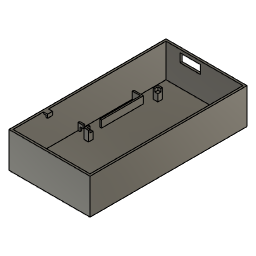
casing (Autodesk Fusion 360 design; units mm, degrees)
Autodesk Fusion 360 part; units mm, degrees
sketch "Sketch1" plane through (0, 0, 0) normal (0, 0, 1) x (1, 0, 0)
  line L0 (-40, 77.5) -> (40, 77.5)
  line L1 (40, 77.5) -> (40, -77.5)
  line L2 (40, -77.5) -> (-40, -77.5)
  line L3 (-40, -77.5) -> (-40, 77.5)
  dimension "d5" = 80
  dimension "d6" = 40
  dimension "d7" = 155
  dimension "d8" = 77.5
  constraint horizontal L0
  constraint vertical L1
  constraint horizontal L2
  constraint vertical L3
  measures "d5" distance of L0.start L0.end
  measures "d6" horizontal distance of origin L0.start
  measures "d7" distance of L0.start L2.end
  measures "d8" vertical distance of origin L0.start
extrude "Extrude1" add sketch "Sketch1" along normal blind 35
shell "Shell1" thickness 2 removed faces 1 at (-13.3333, -25.8333, 35)
sketch "Sketch2" plane through (0, 0, 2) normal (0, 0, 1) x (-1, 0, 0)
  line L0 (38, 75.5) -> (-38, 75.5)
  line L1 (-38, 75.5) -> (-38, -75.5)
  line L2 (-38, -75.5) -> (38, -75.5)
  line L3 (38, -75.5) -> (38, 75.5)
  line L4 (26, -55.5) -> (-24, -55.5)
  line L5 (-24, -55.5) -> (-24, 14.5)
  line L6 (-24, 14.5) -> (26, 14.5)
  line L7 (26, 14.5) -> (26, -55.5)
  line L8 (38, -42.2) -> (30, -42.2)
  line L9 (30, -42.2) -> (30, 9.8)
  line L10 (30, 9.8) -> (38, 9.8)
  line L11 (38, 9.8) -> (38, -42.2)
  line L12 (-28, -75) -> (-33, -75)
  line L13 (-33, -75) -> (-33, 35)
  line L14 (-33, 35) -> (-28, 35)
  line L15 (-28, 35) -> (-28, -75)
  line L16 (-24, 42) -> (-37, 42)
  line L17 (-37, 42) -> (-37, 72)
  line L18 (-37, 72) -> (-24, 72)
  line L19 (-24, 72) -> (-24, 42)
  spline S0 degree 5 poles (-24, 42) (-24.0273, 41.9316) (-24.0869, 41.788) (-24.1914, 41.5521) (-24.3612, 41.196) (-24.6275, 40.6777) (-24.9511, 40.0815) (-25.3338, 39.405) (-25.7728, 38.652) (-26.2629, 37.8296) (-26.7987, 36.9452) (-27.2602, 36.1929) (-27.6235, 35.6054) (-27.8733, 35.2035) (-28, 35) knots 0 0 0 0 0 0 0.1 0.2 0.3 0.4 0.5 0.6 0.7 0.8 0.9 1 1 1 1 1 1
  spline S1 degree 5 poles (-33, 35) (-33.1102, 35.2086) (-33.3283, 35.6201) (-33.648, 36.2209) (-34.0595, 36.9881) (-34.547, 37.8867) (-35.005, 38.718) (-35.4298, 39.4743) (-35.8182, 40.1481) (-36.1686, 40.7356) (-36.4823, 41.24) (-36.7056, 41.5808) (-36.8584, 41.8031) (-36.9539, 41.9368) (-37, 42) knots 0 0 0 0 0 0 0.1 0.2 0.3 0.4 0.5 0.6 0.7 0.8 0.9 1 1 1 1 1 1
  line L20 (-24, 72) -> (0, 72)
  line L21 (0, 72) -> (0, 59)
  line L22 (0, 59) -> (-24, 59)
  line L23 (-24, 59) -> (-24, 72)
  line L24 (0, 62.45) -> (7.5, 62.45)
  line L25 (7.5, 62.45) -> (7.5, 68.55)
  line L26 (7.5, 68.55) -> (0, 68.55)
  line L27 (0, 68.55) -> (0, 62.45)
  line L28 (7.5, 72.95) -> (7.5, 62.45)
  line L29 (7.5, 61.75) -> (11.5, 61.75)
  line L30 (11.5, 61.75) -> (11.5, 69.25)
  line L31 (11.5, 69.25) -> (7.5, 69.25)
  line L32 (7.5, 69.25) -> (7.5, 61.75)
  line L33 (-26.5, -75.5) -> (-28, -75.5)
  line L34 (-28, -75.5) -> (-28, 24.5)
  line L35 (-28, 24.5) -> (-26.5, 24.5)
  line L36 (-26.5, 24.5) -> (-26.5, -75.5)
  line L37 (-33, -75.5) -> (-34.5, -75.5)
  line L38 (-34.5, -75.5) -> (-34.5, 24.5)
  line L39 (-34.5, 24.5) -> (-33, 24.5)
  line L40 (-33, 24.5) -> (-33, -75.5)
  line L41 (-24, 59) -> (1.5, 59)
  line L42 (1.5, 59) -> (1.5, 57.5)
  line L43 (1.5, 57.5) -> (-24, 57.5)
  line L44 (-24, 57.5) -> (-24, 59)
  line L45 (0, 59) -> (1.5, 59)
  line L46 (1.5, 59) -> (1.5, 61)
  line L47 (1.5, 61) -> (0, 61)
  line L48 (0, 61) -> (0, 59)
  line L49 (-24, 57.5) -> (-22.5, 57.5)
  line L50 (-22.5, 57.5) -> (-22.5, 45)
  line L51 (-22.5, 45) -> (-24, 45)
  line L52 (-24, 45) -> (-24, 57.5)
  line L53 (26, -55.5) -> (23, -55.5)
  line L54 (23, -55.5) -> (23, -52.5)
  line L55 (23, -52.5) -> (26, -52.5)
  line L56 (26, -52.5) -> (26, -55.5)
  line L57 (-24, -55.5) -> (-21, -55.5)
  line L58 (-21, -55.5) -> (-21, -52.5)
  line L59 (-21, -52.5) -> (-24, -52.5)
  line L60 (-24, -52.5) -> (-24, -55.5)
  line L61 (23, -55.5) -> (26, -55.5)
  line L62 (26, -55.5) -> (26, -57)
  line L63 (26, -57) -> (23, -57)
  line L64 (23, -57) -> (23, -55.5)
  line L65 (26, -57) -> (27.5, -57)
  line L66 (27.5, -57) -> (27.5, -52.5)
  line L67 (27.5, -52.5) -> (26, -52.5)
  line L68 (26, -52.5) -> (26, -57)
  line L69 (-21, -55.5) -> (-24, -55.5)
  line L70 (-24, -55.5) -> (-24, -57)
  line L71 (-24, -57) -> (-21, -57)
  line L72 (-21, -57) -> (-21, -55.5)
  line L73 (-24, -57) -> (-25.5, -57)
  line L74 (-25.5, -57) -> (-25.5, -52.5)
  line L75 (-25.5, -52.5) -> (-24, -52.5)
  line L76 (-24, -52.5) -> (-24, -57)
  line L77 (38, -42.2) -> (28.5, -42.2)
  line L78 (28.5, -42.2) -> (28.5, -43.7)
  line L79 (28.5, -43.7) -> (38, -43.7)
  line L80 (38, -43.7) -> (38, -42.2)
  line L81 (30, -42.2) -> (28.5, -42.2)
  line L82 (28.5, -42.2) -> (28.5, -2.2)
  line L83 (28.5, -2.2) -> (30, -2.2)
  line L84 (30, -2.2) -> (30, -42.2)
  line L85 (38, 9.8) -> (33, 9.8)
  line L86 (33, 9.8) -> (33, 11.3)
  line L87 (33, 11.3) -> (38, 11.3)
  line L88 (38, 11.3) -> (38, 9.8)
  line L89 (26, 14.5) -> (23, 14.5)
  line L90 (23, 14.5) -> (23, 11.5)
  line L91 (23, 11.5) -> (26, 11.5)
  line L92 (26, 11.5) -> (26, 14.5)
  line L93 (26, 11.5) -> (27.5, 11.5)
  line L94 (27.5, 11.5) -> (27.5, 16)
  line L95 (27.5, 16) -> (26, 16)
  line L96 (26, 16) -> (26, 11.5)
  line L97 (26, 14.5) -> (23, 14.5)
  line L98 (23, 14.5) -> (23, 16)
  line L99 (23, 16) -> (26, 16)
  line L100 (26, 16) -> (26, 14.5)
  line L101 (-24, 14.5) -> (-21, 14.5)
  line L102 (-21, 14.5) -> (-21, 11.5)
  line L103 (-21, 11.5) -> (-24, 11.5)
  line L104 (-24, 11.5) -> (-24, 14.5)
  line L105 (-21, 14.5) -> (-25.5, 14.5)
  line L106 (-25.5, 14.5) -> (-25.5, 16)
  line L107 (-25.5, 16) -> (-21, 16)
  line L108 (-21, 16) -> (-21, 14.5)
  line L109 (-24, 14.5) -> (-25.5, 14.5)
  line L110 (-25.5, 14.5) -> (-25.5, 11.5)
  line L111 (-25.5, 11.5) -> (-24, 11.5)
  line L112 (-24, 11.5) -> (-24, 14.5)
  line L113 (-24, 75.5) -> (0, 75.5)
  line L114 (0, 75.5) -> (0, 72.5)
  line L115 (0, 72.5) -> (-24, 72.5)
  line L116 (-24, 72.5) -> (-24, 75.5)
  line L117 (0, 75.5) -> (1.5, 75.5)
  line L118 (1.5, 75.5) -> (1.5, 70)
  line L119 (1.5, 70) -> (0, 70)
  line L120 (0, 70) -> (0, 75.5)
  point P0 (-25, 40)
  point P1 (-35.7549, 40.0344)
  dimension "d12" = 50
  dimension "d13" = 70
  dimension "d14" = 20
  dimension "d15" = 12
  dimension "d16" = 8
  dimension "d17" = 52
  dimension "d18" = 110
  dimension "d19" = 5
  dimension "d20" = 13
  dimension "d21" = 30
  dimension "d22" = 0.5
  dimension "d23" = 1
  dimension "d24" = 7
  dimension "d25" = 5
  dimension "d26" = 24
  dimension "d27" = 13
  dimension "d28" = 7.5
  dimension "d29" = 6.1
  dimension "d32" = 3.45
  dimension "d33" = 7.5
  dimension "d34" = 4
  dimension "d35" = 2.75
  dimension "d36" = 1.5
  dimension "d37" = 100
  dimension "d38" = 1.5
  dimension "d39" = 100
  dimension "d40" = 3.5
  dimension "d41" = 25.5
  dimension "d42" = 1.5
  dimension "d43" = 2
  dimension "d44" = 1.5
  dimension "d45" = 12.5
  dimension "d46" = 1.5
  dimension "d47" = 13.3
  dimension "d48" = 3
  dimension "d49" = 3
  dimension "d50" = 3
  dimension "d51" = 3
  dimension "d52" = 1.5
  dimension "d53" = 3
  dimension "d54" = 1.5
  dimension "d55" = 4.5
  dimension "d56" = 3
  dimension "d57" = 1.5
  dimension "d58" = 1.5
  dimension "d59" = 4.5
  dimension "d60" = 4
  dimension "d61" = 1.5
  dimension "d62" = 9.5
  dimension "d63" = 40
  dimension "d64" = 1.5
  dimension "d65" = 5
  dimension "d66" = 1.5
  dimension "d67" = 3
  dimension "d68" = 3
  dimension "d69" = 1.5
  dimension "d70" = 4.5
  dimension "d71" = 3
  dimension "d72" = 1.5
  dimension "d73" = 3
  dimension "d74" = 3
  dimension "d75" = 1.5
  dimension "d76" = 4.5
  dimension "d77" = 1.5
  dimension "d78" = 3
  dimension "d85" = 13
  dimension "d86" = 3
  dimension "d87" = 24
  dimension "d88" = 1.5
  dimension "d89" = 5.5
  constraint horizontal L4
  constraint vertical L5
  constraint horizontal L6
  constraint vertical L7
  constraint horizontal L8
  constraint vertical L9
  constraint horizontal L10
  constraint vertical L11
  constraint horizontal L12
  constraint vertical L13
  constraint horizontal L14
  constraint vertical L15
  constraint horizontal L16
  constraint vertical L17
  constraint horizontal L18
  constraint vertical L19
  constraint horizontal L20
  constraint vertical L21
  constraint horizontal L22
  constraint vertical L23
  constraint horizontal L24
  constraint vertical L25
  constraint horizontal L26
  constraint vertical L27
  constraint coincident L21 L24.start
  constraint vertical L28
  constraint horizontal L29
  constraint vertical L30
  constraint horizontal L31
  constraint vertical L32
  constraint horizontal L33
  constraint vertical L34
  constraint horizontal L35
  constraint vertical L36
  constraint coincident L15 L34.end
  constraint coincident L2 L33.start
  constraint horizontal L37
  constraint vertical L38
  constraint horizontal L39
  constraint vertical L40
  constraint coincident L2 L37.start
  constraint horizontal L41
  constraint vertical L42
  constraint horizontal L43
  constraint vertical L44
  constraint horizontal L45
  constraint vertical L46
  constraint horizontal L47
  constraint vertical L48
  constraint horizontal L49
  constraint vertical L50
  constraint horizontal L51
  constraint vertical L52
  constraint horizontal L53
  constraint vertical L54
  constraint horizontal L55
  constraint vertical L56
  constraint horizontal L57
  constraint vertical L58
  constraint horizontal L59
  constraint vertical L60
  constraint horizontal L61
  constraint vertical L62
  constraint horizontal L63
  constraint vertical L64
  constraint horizontal L65
  constraint vertical L66
  constraint horizontal L67
  constraint vertical L68
  constraint horizontal L69
  constraint vertical L70
  constraint horizontal L71
  constraint vertical L72
  constraint horizontal L73
  constraint vertical L74
  constraint horizontal L75
  constraint vertical L76
  constraint horizontal L77
  constraint vertical L78
  constraint horizontal L79
  constraint vertical L80
  constraint horizontal L81
  constraint vertical L82
  constraint horizontal L83
  constraint vertical L84
  constraint horizontal L85
  constraint vertical L86
  constraint horizontal L87
  constraint vertical L88
  constraint horizontal L89
  constraint vertical L90
  constraint horizontal L91
  constraint vertical L92
  constraint horizontal L93
  constraint vertical L94
  constraint horizontal L95
  constraint vertical L96
  constraint horizontal L97
  constraint vertical L98
  constraint horizontal L99
  constraint vertical L100
  constraint horizontal L101
  constraint vertical L102
  constraint horizontal L103
  constraint vertical L104
  constraint horizontal L105
  constraint vertical L106
  constraint horizontal L107
  constraint vertical L108
  constraint horizontal L109
  constraint vertical L110
  constraint horizontal L111
  constraint vertical L112
  constraint horizontal L113
  constraint vertical L114
  constraint horizontal L115
  constraint vertical L116
  constraint coincident L0 L113.start
  constraint horizontal L117
  constraint vertical L118
  constraint horizontal L119
  constraint vertical L120
  measures "d12" distance of L4.start L4.end
  measures "d13" distance of L4.start L6.end
  measures "d14" distance of L2 L4.start
  measures "d15" horizontal distance of L2.end L6.end
  measures "d16" distance of L8.start L8.end
  measures "d17" distance of L8.start L10.end
  measures "d18" distance of L12.end L13.end
  measures "d19" distance of L12.start L12.end
  measures "d20" distance of L16.start L16.end
  measures "d21" distance of L16.start L18.end
  measures "d22" distance of L2 L12.start
  measures "d23" horizontal distance of L0.end L16.end
  measures "d24" vertical distance of L14.end L16.start
  measures "d25" distance of L1 L13.end
  measures "d26" distance of L21.end L22.end
  measures "d27" distance of L20.end L21.end
  measures "d28" distance of L24.start L24.end
  measures "d29" distance of L24.end L25.end
  measures "d32" distance of L20.end L26.end
  measures "d33" distance of L29.end L30.end
  measures "d34" distance of L29.start L29.end
  measures "d35" vertical distance of L20.end L30.end
  measures "d36" distance of L33.start L33.end
  measures "d37" distance of L33.start L35.end
  measures "d38" distance of L37.start L37.end
  measures "d39" distance of L37.end L38.end
  measures "d40" distance of L1.end L37.end
  measures "d41" distance of L42.end L43.end
  measures "d42" distance of L41.end L42.end
  measures "d43" distance of L41.end L46.end
  measures "d44" distance of L21.end L41.end
  measures "d45" distance of L49.end L50.end
  measures "d46" distance of L50.end L51.end
  measures "d47" vertical distance of L4.start L8.start
  measures "d48" distance of L4.start L53.end
  measures "d49" distance of L4.start L55.end
  measures "d50" distance of L4.end L57.end
  measures "d51" distance of L4.end L59.end
  measures "d52" distance of L53.end L63.end
  measures "d53" distance of L53.end L4.start
  measures "d54" distance of L62.end L65.end
  measures "d55" distance of L65.end L66.end
  measures "d56" distance of L70.end L71.end
  measures "d57" distance of L4.end L70.end
  measures "d58" distance of L70.end L73.end
  measures "d59" distance of L70.end L59.end
  measures "d60" distance of L7 L8.end
  measures "d61" distance of L8.start L79.end
  measures "d62" distance of L8.start L77.end
  measures "d63" distance of L77.end L82.end
  measures "d64" distance of L82.end L83.end
  measures "d65" distance of L10.end L85.end
  measures "d66" distance of L10.end L87.end
  measures "d67" distance of L90.end L91.end
  measures "d68" distance of L89.end L90.end
  measures "d69" distance of L91.end L93.end
  measures "d70" distance of L93.end L94.end
  measures "d71" distance of L98.end L95.end
  measures "d72" distance of L89.end L98.end
  measures "d73" distance of L102.end L103.end
  measures "d74" distance of L101.end L102.end
  measures "d75" distance of L101.end L107.end
  measures "d76" distance of L106.end L107.end
  measures "d77" distance of L103.end L110.end
  measures "d78" distance of L105.end L110.end
  measures "d85" horizontal distance of L17.end L113.start
  measures "d86" distance of L113.start L115.end
  measures "d87" distance of L113.start L113.end
  measures "d88" distance of L113.end L117.end
  measures "d89" distance of L117.end L118.end
extrude "Extrude2" add sketch "Sketch2" along normal blind 7 contours L2 L13 L37 L38 L39 L40 | L19 L22 L41 L42 L43 L44 L45 L49 | L21 L41 L45 L46 L47 L48 | L2 L15 L33 L34 L35 L36 | L19 L43 L49 L50 L51 L52
extrude "Extrude3" add sketch "Sketch2" along normal blind 7 contours L4 L7 L53 L54 L55 L56 L61 L68 | L4 L5 L57 L58 L59 L60 L69 L76 | L6 L7 L89 L90 L91 L92 L96 L97 | L5 L6 L101 L102 L103 L104 L105 L112
extrude "Extrude4" add sketch "Sketch2" along normal blind 10 contours L4 L53 L61 L62 L63 L64 L68 | L7 L56 L62 L65 L66 L67 L68 | L4 L57 L69 L70 L71 L72 L76 | L7 L92 L93 L94 L95 L96 L100 | L5 L60 L70 L73 L74 L75 L76 | L6 L89 L96 L97 L98 L99 L100 | L5 L104 L105 L109 L110 L111 L112 | L6 L101 L105 L106 L107 L108 L109
extrude "Extrude5" add sketch "Sketch2" along normal blind 7 contours L0 L21 L114 L117 L118 L119 L120 | L0 L113 L114 L115 L116 L120
extrude "Extrude6" add sketch "Sketch2" along normal blind 7 contours L3 L10 L85 L86 L87 L88 | L3 L8 L77 L78 L79 L80 L81 | L9 L77 L81 L82 L83 L84
sketch "Sketch3" plane through (0, 75.5, 0) normal (0, -1, 0) x (1, 0, 0)
  line L0 (34.5, 9) -> (34.5, 2)
  line L1 (34.5, 2) -> (38, 2)
  line L2 (38, 2) -> (38, 35)
  line L3 (38, 35) -> (-38, 35)
  line L4 (-38, 35) -> (-38, 2)
  line L5 (-38, 2) -> (26.5, 2)
  line L6 (26.5, 2) -> (26.5, 9)
  line L7 (26.5, 9) -> (28, 9)
  line L8 (28, 9) -> (28, 2)
  line L9 (28, 2) -> (33, 2)
  line L10 (33, 2) -> (33, 9)
  line L11 (33, 9) -> (34.5, 9)
  line L12 (-24, 32) -> (-4, 32)
  line L13 (-4, 32) -> (-4, 23.5)
  line L14 (-4, 23.5) -> (-24, 23.5)
  line L15 (-24, 23.5) -> (-24, 32)
  point P0 (-40, 35)
  point P1 (-40, 0)
  dimension "d94" = 8.5
  dimension "d95" = 20
  dimension "d96" = 16
  dimension "d97" = 23.5
  constraint horizontal L12
  constraint vertical L13
  constraint horizontal L14
  constraint vertical L15
  measures "d94" distance of L12.start L14.end
  measures "d95" distance of L13.end L14.end
  measures "d96" horizontal distance of L14.end P0
  measures "d97" vertical distance of L14.end P1
extrude "Extrude7" cut sketch "Sketch3" against normal blind 2 contours L12 L13 L14 L15
sketch "Sketch4" plane through (0, -11.3, 0) normal (0, -1, 0) x (1, 0, 0)
  line L0 (-38, 2) -> (-33, 2)
  line L1 (-33, 2) -> (-33, 9)
  line L2 (-33, 9) -> (-38, 9)
  line L3 (-38, 9) -> (-38, 2)
  line L4 (-33, 2) -> (-36, 2)
  line L5 (-36, 2) -> (-36, 6)
  line L6 (-36, 6) -> (-33, 6)
  line L7 (-33, 6) -> (-33, 2)
  dimension "d100" = 3
  dimension "d101" = 4
  constraint horizontal L4
  constraint vertical L5
  constraint horizontal L6
  constraint vertical L7
  constraint coincident L0.end L1.start
  measures "d100" distance of L5.end L6.end
  measures "d101" distance of L0.end L6.end
extrude "Extrude8" cut sketch "Sketch4" against normal blind 1.5 contours L0 L1 L4 L5 L6 L7
sketch "Sketch5" plane through (-38, 0, 0) normal (1, 0, 0) x (0, 1, 0)
  line L0 (-9.8, 9) -> (-9.8, 2)
  line L1 (-9.8, 2) -> (42.2, 2)
  line L2 (42.2, 2) -> (42.2, 9)
  line L3 (42.2, 9) -> (43.7, 9)
  line L4 (43.7, 9) -> (43.7, 2)
  line L5 (43.7, 2) -> (75.5, 2)
  line L6 (75.5, 2) -> (75.5, 35)
  line L7 (75.5, 35) -> (-75.5, 35)
  line L8 (-75.5, 35) -> (-75.5, 2)
  line L9 (-75.5, 2) -> (-11.3, 2)
  line L10 (-11.3, 2) -> (-11.3, 9)
  line L11 (-11.3, 9) -> (-9.8, 9)
  line L12 (-45.5, 35) -> (-40.5, 35)
  line L13 (-40.5, 35) -> (-40.5, 33.5)
  line L14 (-40.5, 33.5) -> (-45.5, 33.5)
  line L15 (-45.5, 33.5) -> (-45.5, 35)
  point P0 (-77.5, 35)
  dimension "d104" = 32
  dimension "d105" = 5
  dimension "d106" = 1.5
  constraint horizontal L12
  constraint vertical L13
  constraint horizontal L14
  constraint vertical L15
  constraint coincident L7 L12.start
  measures "d104" distance of L12.start P0
  measures "d105" distance of L12.start L12.end
  measures "d106" distance of L12.start L14.end
extrude "Extrude9" add sketch "Sketch5" along normal blind 4 contours L7 L12 L13 L14 L15
sketch "Sketch6" plane through (0, 0, 33.5) normal (0, 0, -1) x (1, 0, 0)
  line L0 (-38, 45.5) -> (-38, 40.5)
  line L1 (-38, 40.5) -> (-34, 40.5)
  line L2 (-34, 40.5) -> (-34, 45.5)
  line L3 (-34, 45.5) -> (-38, 45.5)
  line L4 (-34, 40.5) -> (-35.5, 40.5)
  line L5 (-35.5, 40.5) -> (-35.5, 45.5)
  line L6 (-35.5, 45.5) -> (-34, 45.5)
  line L7 (-34, 45.5) -> (-34, 40.5)
  dimension "d109" = 1.5
  constraint horizontal L4
  constraint vertical L5
  constraint horizontal L6
  constraint vertical L7
  constraint coincident L3 L5.end
  constraint coincident L1.end L2.start
  measures "d109" distance of L1.end L4.end
extrude "Extrude10" add sketch "Sketch6" along normal blind 2 contours L1 L2 L3 L4 L5 L6 L7
